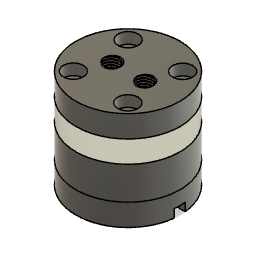
main_sensor_holder (Autodesk Fusion 360 design; units mm, degrees)
Autodesk Fusion 360 part; units mm, degrees
sketch "body_sketch" plane through (0, 0, 0) normal (0, 1, 0) x (1, 0, 0)
  circle A0 centre (0, 0) radius 19
  circle A1 centre (0, 0) radius 9.25
  circle A2 centre (0, 0) radius 14.125 construction
  circle A3 centre (9.9532, -10.0225) radius 1.65
  circle A4 centre (10.0225, 9.9532) radius 1.65
  circle A5 centre (-9.9532, 10.0225) radius 1.65
  circle A6 centre (-10.0225, -9.9532) radius 1.65
  circle A7 centre (0, 0) radius 8.25
  circle A8 centre (0, 0) radius 9.15
  circle A9 centre (9.9532, -10.0225) radius 2.1
  circle A10 centre (10.0225, 9.9532) radius 2.1
  circle A11 centre (-9.9532, 10.0225) radius 2.1
  circle A12 centre (-10.0225, -9.9532) radius 2.1
  dimension "screws_ring_dia" = 28.25
  dimension "body_dia" = 38
  dimension "sensor_cavity_dia" = 18.5
  dimension "screw_thread_hole_dia" = 3.3
  dimension "d12" = 360
  dimension "sensor_rim_min_dia" = 16.5
  dimension "sensor_holding_cylinder_clearance" = 18.3
  dimension "screw_through_hole_dia" = 4.2
  dimension "d70" = 360
  constraint coincident A0.centre A1.centre
  constraint concentric A0 A2
  constraint coincident A2 A3.centre
  constraint concentric A1 A7
  constraint concentric A1 A8
  constraint concentric A3 A9
  measures "screws_ring_dia" diameter of A2
  measures "body_dia" diameter of A0
  measures "sensor_cavity_dia" diameter of A1
  measures "screw_thread_hole_dia" diameter of A3
  measures "sensor_rim_min_dia" diameter of A7
  measures "sensor_holding_cylinder_clearance" diameter of A8
  measures "screw_through_hole_dia" diameter of A9
extrude "Extrude1" add sketch "body_sketch" along normal blind 12 contours A0 | A9 | A10 | A11 | A12 makes body 1
ref_plane "WorkPlane1" through (0, 12, 0) normal (0, 1, 0) x (1, 0, 0)
sketch " ptfe_disc_sketch_sensor_side" plane through (0, 12, 0) normal (0, 1, 0) x (1, 0, 0)
  circle A0 centre (0, 0) radius 2
  circle A1 centre (-9.9532, 10.0225) radius 2.1
  circle A2 centre (0, 0) radius 9.25
  circle A3 centre (0, 0) radius 19
  circle A4 centre (0, 0) radius 2.5 construction
  circle A5 centre (2.5, 0) radius 0.5
  circle A6 centre (-2.5, 0) radius 0.5
  line L0 (-9.9532, 10.0225) -> (10.3055, -10.3772) construction
  line L1 (0, 0) -> (-2.5, 0) construction
  circle A7 centre (0, 0) radius 14.125 construction
  circle A8 centre (-10.0225, -9.9532) radius 2.1
  circle A9 centre (9.9532, -10.0225) radius 2.1
  circle A10 centre (10.0225, 9.9532) radius 2.1
  point P0 (-9.9532, 10.0225)
  dimension "fluid_chann_intern_dist" = 5
  dimension "fluid_channel_dia" = 1
  dimension "d23" = 360
  dimension "d28" = 360
  dimension "PTFE_disc_screw_hole_dia" = 4.2
  constraint coincident A0.centre A2.centre
  constraint coincident A4 A5.centre
  constraint coincident P0 A1.centre
  constraint coincident A6.centre L1.end
  constraint concentric A0 A7
  measures "fluid_chann_intern_dist" diameter of A4
  measures "fluid_channel_dia" diameter of A5
  measures "PTFE_disc_screw_hole_dia" diameter of A1
extrude "Extrude3" add sketch " ptfe_disc_sketch_sensor_side" along normal blind 8 separate body contours A0 | A6 | A5 | A2 | A3 makes body 2
ref_plane "WorkPlane2" through (0, 20, 0) normal (0, 1, 0) x (1, 0, 0)
sketch "ptfe_disc_inlet_side" plane through (0, 20, 0) normal (0, 1, 0) x (1, 0, 0)
  circle A0 centre (0, 0) radius 6 construction
  circle A1 centre (-6, 0) radius 0.5
  circle A2 centre (6, 0) radius 0.5
  circle A3 centre (0, 0) radius 19
  circle A4 centre (-9.9532, 10.0225) radius 2.1
  circle A5 centre (-10.0225, -9.9532) radius 2.1
  circle A6 centre (9.9532, -10.0225) radius 2.1
  circle A7 centre (10.0225, 9.9532) radius 2.1
  circle A8 centre (-6, 0) radius 2
  circle A9 centre (6, 0) radius 2
  point P0 (-2.5, 0)
  point P1 (2.5, 0)
  point P2 (-9.9532, 10.0225)
  point P3 (-10.0225, -9.9532)
  point P4 (10.3055, -10.3772)
  point P5 (10.0225, 9.9532)
  dimension "fluid_channel_dia_inlet" = 1
  dimension "d35" = 360
  dimension "fluid_channel_inlet_dist" = 12
  dimension "d37" = 4.2
  dimension "d39" = 360
  dimension "fluidid_connectors_dia" = 4
  dimension "d42" = 360
  constraint coincident A0.centre A3.centre
  constraint coincident A0 A1.centre
  constraint collinear P0 A0.centre A1.centre
  constraint coincident P2 A4.centre
  constraint concentric A1 A8
  measures "fluid_channel_dia_inlet" diameter of A1
  measures "fluid_channel_inlet_dist" diameter of A0
  measures "d37" diameter of A4
  measures "fluidid_connectors_dia" diameter of A8
loft "Loft1" cut profiles " ptfe_disc_sketch_sensor_side", "ptfe_disc_inlet_side" section 1 contours A6 section 2 contours A1 bodies 2
loft "Loft2" cut profiles " ptfe_disc_sketch_sensor_side", "ptfe_disc_inlet_side" section 1 contours A5 section 2 contours A2 bodies 2
extrude "Extrude4" add sketch "ptfe_disc_inlet_side" along normal blind 8 separate body contours A3 makes body 3
copy_body "Body->Comp1" bodies 2 removing the originals makes body 4 in component "PTFE_disc"
copy_body "Body->Comp2" bodies 3 removing the originals makes body 5 in component "top_holder"
extrude "Extrude1'" add sketch "body_sketch" against normal blind 8 separate body contours A0 | A1 | A8 makes body 6 in component "bottom_sensor_holder"
extrude "Extrude3'" add sketch "body_sketch" along normal blind 4.8 contours A8 bodies 6 in component "bottom_sensor_holder"
ref_plane "WorkPlane4" through (0, 28, 0) normal (0, 1, 0) x (1, 0, 0)
sketch "top_face_sketch" plane through (0, 28, 0) normal (0, 1, 0) x (1, 0, 0)
  circle A0 centre (0, 0) radius 19
  circle A1 centre (-9.9532, 10.0225) radius 3.65
  circle A2 centre (-10.0225, -9.9532) radius 3.65
  circle A3 centre (9.9532, -10.0225) radius 3.65
  circle A4 centre (10.0225, 9.9532) radius 3.65
  point P0 (-9.9532, 10.0225)
  point P1 (10.0225, 9.9532)
  point P2 (9.9532, -10.0225)
  point P3 (-10.0225, -9.9532)
  dimension "screw_head_counter_bore" = 7.3
  dimension "d65" = 360
  constraint coincident P0 A1.centre
  measures "screw_head_counter_bore" diameter of A1
extrude "Extrude1''" cut sketch "top_face_sketch" against normal blind 4 contours A1 | A2 | A3 | A4 bodies 5 in component "top_holder"
ref_plane "WorkPlane5" through (0, -8, 0) normal (0, -1, 0) x (-1, 0, 0)
sketch "bottom_face_sketch" plane through (0, -8, 0) normal (0, -1, 0) x (1, 0, 0)
  circle A0 centre (9.9532, 10.0225) radius 2.1
  circle A1 centre (10.0225, -9.9532) radius 2.1
  circle A2 centre (-10.0225, 9.9532) radius 2.1
  circle A3 centre (-9.9532, -10.0225) radius 2.1
  circle A4 centre (0, 0) radius 8.25
  circle A5 centre (0, 0) radius 19
  circle A6 centre (-10.0225, 9.9532) radius 3.65
  circle A7 centre (-9.9532, -10.0225) radius 3.65
  circle A8 centre (10.0225, -9.9532) radius 3.65
  circle A9 centre (9.9532, 10.0225) radius 3.65
  line L0 (10.0225, -9.9532) -> (-9.9532, -10.0225) construction
  line L1 (-10.0225, 9.9532) -> (9.9532, 10.0225) construction
  circle A10 centre (-0.0473, 13.6249) radius 1.25
  line L2 (-0.0659, 18.9999) -> (-0.0286, 8.25) construction
  line L3 (-0.0473, 13.6249) -> (-10.0225, 9.9532) construction
  line L4 (-0.0473, 13.6249) -> (9.9532, 10.0225) construction
  circle A11 centre (-13.6249, -0.0473) radius 1.25
  line L5 (8.0039, -2) -> (18.8944, -2)
  line L6 (0, 0) -> (19, 0) construction
  line L7 (8.0039, 2) -> (18.8944, 2)
  circle A12 centre (0.0473, -13.6249) radius 1.25
  circle A13 centre (13.6249, 0.0473) radius 1.25
  point P0 (-10.0225, 9.9532)
  point P1 (-9.9532, -10.0225)
  point P2 (10.0225, -9.9532)
  point P3 (9.9532, 10.0225)
  dimension "screw_head_bore_bottom_dia" = 7.3
  dimension "d74" = 360
  dimension "mounting_screw_thread_hole" = 2.5
  dimension "d81" = 360
  dimension "cable_channel_width" = 2
  constraint coincident P0 A2.centre
  constraint coincident A1.centre A8.centre
  constraint coincident P1 A3.centre
  constraint coincident P3 A0.centre
  constraint coincident A10.centre L2
  constraint perpendicular L1 L2
  constraint coincident A10.centre L3.start
  constraint equal L3 L4
  constraint coincident A5 L2.start
  constraint coincident A4 L2.end
  constraint midpoint A10.centre L2
  constraint horizontal L5
  constraint coincident A4.centre A5.centre
  constraint coincident A5 L6.end
  constraint horizontal L6
  constraint symmetric L5.end L6 L7.end
  constraint symmetric L5.start L6 L7.start
  constraint coincident A4 L5.start
  constraint coincident A5 L5.end
  measures "screw_head_bore_bottom_dia" diameter of A6
  measures "mounting_screw_thread_hole" diameter of A10
  measures "cable_channel_width" distance of L5 L6
extrude "Extrude4'" cut sketch "bottom_face_sketch" against normal blind 4.6 contours A6 | A7 | A8 | A9 bodies 6 in component "bottom_sensor_holder"
extrude "Extrude5" cut sketch "bottom_face_sketch" against normal blind 3 contours A4 A5 L5 L7 | A13 picked at (13.4766, -1.7331) bodies 6 in component "bottom_sensor_holder"
extrude "Extrude6" cut sketch "bottom_face_sketch" against normal blind 8 contours A10 | A11 | A12 bodies 6 in component "bottom_sensor_holder"
thread "Thread1" "ANSI Unified Screw Threads 0.25 1/4-28 UNF 1B" major diameter 6.35 minor diameter 5.4737 pitch 0.9071 angle 60 modelled right hand crest width 0.2395 on face at (-4.0099, 22.6667, 0.1991) crest through (-3.2632, 20.2268, 0) on face at (7.9901, 22.6667, 0.1991) crest through (8.7369, 20.2268, 0) on bodies 5 in component "top_holder"
thread "Thread1'" "ISO Metric profile 4.0 M4x0.7 6H" major diameter 4.1095 minor diameter 3.332 pitch 0.7 angle 60 modelled right hand crest width 0.193 on face at (-8.3745, 8, 10.0354) crest through (-8.3565, 0.175, 9.9532) on face at (11.6011, 8, 10.1047) crest through (11.6192, 0.175, 10.0225) on face at (11.6704, 8, -9.8709) crest through (11.6885, 0.175, -9.9532) on face at (-8.3052, 8, -9.9402) crest through (-8.2872, 0.175, -10.0225) on bodies 1
thread "Thread1''" "ISO Metric profile 3.0 M3x0.5 6H" major diameter 3.086 minor diameter 2.529 pitch 0.5 angle 60 modelled right hand crest width 0.1368 on face at (1.1965, -2.6667, 13.5005) crest through (1.2172, -7.875, 13.6249) on face at (-12.3811, -2.6667, -0.1717) crest through (-13.6249, -7.875, 1.2172) on face at (1.291, -2.6667, -13.7494) crest through (1.3118, -7.875, -13.6249) on bodies 6 in component "bottom_sensor_holder"
ref_plane "WorkPlane1" through (0, 12, 0) normal (0, -1, 0) x (-1, 0, 0) in component "centering_ring"
sketch "Sketch1" plane through (0, 12, 0) normal (0, -1, 0) x (1, 0, 0) in component "centering_ring"
  circle A0 centre (0, 0) radius 9.25
  circle A1 centre (0, 0) radius 9.15
  circle A2 centre (0, 0) radius 7.25
  dimension "centering_ring_outside_dia" = 18.3
  dimension "centering_ring_inside_dia" = 14.5
  constraint concentric A0 A1
  constraint concentric A0 A2
  measures "centering_ring_outside_dia" diameter of A1
  measures "centering_ring_inside_dia" diameter of A2
extrude "Extrude1'''" add sketch "Sketch1" along normal blind 0.8 separate body contours A1 makes body 7 in component "centering_ring"
ref_plane "WorkPlane1" through (-0.0528, -8, 0) normal (0, -1, 0) x (-1, 0, 0) in component "holding_plate"
sketch "Sketch1 (2)" plane through (-0.0528, -8, 0) normal (0, -1, 0) x (1, 0, 0) in component "holding_plate"
  circle A0 centre (0.0528, 0) radius 19
  circle A1 centre (0.0528, 0) radius 8.25
  circle A2 centre (0.1, -13.6249) radius 1.25
  circle A3 centre (0.0055, 13.6249) radius 1.25
  circle A4 centre (-13.5721, -0.0473) radius 1.25
  line L0 (8.0567, -2) -> (18.9472, -2)
  line L1 (8.0567, 2) -> (18.9472, 2)
  line L2 (0, -25) -> (0.0528, 26.3634) construction
  line L3 (28, 0) -> (-44, 0) construction
  line L4 (0.0062, -18.9999) -> (-39.9938, -18.9999)
  line L5 (-39.9938, -18.9999) -> (-39.9938, 19.0001)
  line L6 (-39.9938, 19.0001) -> (0.0062, 19.0001)
  line L7 (0.0062, 19.0001) -> (0.0062, -18.9999)
  ellipse E0 centre (0.0528, 0) end of major axis (0.0062, -18.9999) minor radius 19
  line L8 (0.0994, 18.9999) -> (0.0062, -18.9999) construction
  line L9 (-18.9472, 0.0466) -> (19.0527, -0.0466) construction
  line L10 (-39.9938, 19.0001) -> (-38.3938, 19.0001)
  line L11 (-38.3938, 19.0001) -> (-38.3938, -18.9999)
  line L12 (-38.3938, -18.9999) -> (-39.9938, -18.9999)
  line L13 (-39.9938, -18.9999) -> (-39.9938, 19.0001)
  dimension "d93" = 40
  dimension "d94" = 38
  dimension "d95" = 1.6
  constraint horizontal L3
  constraint horizontal L4
  constraint vertical L5
  constraint horizontal L6
  constraint vertical L7
  constraint coincident A0 L4.start
  constraint coincident L2 L4.start
  constraint coincident E0 L8.start
  constraint coincident L4.start E0
  constraint coincident E0 L9.start
  constraint coincident E0 L9.end
  constraint concentric A0 E0
  constraint horizontal L10
  constraint vertical L11
  constraint horizontal L12
  constraint vertical L13
  constraint coincident L4 L11.end
  measures "d93" distance of L4.start L4.end
  measures "d94" distance of L4.end L5.end
  measures "d95" distance of L5.end L10.end
ref_plane "WorkPlane1" through (-40, 0, 0) normal (1, 0, 0) x (0, 1, 0) in component "holding_plate"
sketch "Sketch2" plane through (-40, 0, 0) normal (1, 0, 0) x (0, 0, -1) in component "holding_plate"
  line L0 (-19, -8) -> (19, -8)
  line L1 (19, -8) -> (19, 12)
  line L2 (14, 17) -> (-14, 17)
  line L3 (-19, 12) -> (-19, -8)
  line L4 (-14, 17) -> (-19, 12)
  line L5 (19, 12) -> (14, 17)
  line L6 (-19, -8) -> (19, -8)
  line L7 (18.9999, -8) -> (-19.0001, -8)
  line L8 (0, 19) -> (0, -14) construction
  line L9 (-22, 5) -> (23, 5) construction
  line L10 (-13, 13) -> (-5, 13)
  line L11 (-5, 13) -> (-5, 9)
  line L12 (-5, 9) -> (-13, 9)
  line L13 (-13, 9) -> (-13, 13)
  circle A0 centre (-13, 11) radius 2
  circle A1 centre (-5, 11) radius 2
  circle A2 centre (13, 11) radius 2
  circle A3 centre (5, 11) radius 2
  line L14 (13, 13) -> (5, 13)
  line L15 (5, 13) -> (5, 9)
  line L16 (13, 9) -> (13, 13)
  line L17 (5, 9) -> (13, 9)
  line L18 (5, 1) -> (13, 1)
  line L19 (-13, 1) -> (-13, -3)
  circle A4 centre (-13, -1) radius 2
  circle A5 centre (5, -1) radius 2
  line L20 (13, -3) -> (5, -3)
  circle A6 centre (13, -1) radius 2
  line L21 (13, 1) -> (13, -3)
  circle A7 centre (-5, -1) radius 2
  line L22 (-13, -3) -> (-5, -3)
  line L23 (-5, 1) -> (-13, 1)
  line L24 (5, -3) -> (5, 1)
  line L25 (-5, -3) -> (-5, 1)
  point P0 (19, 17)
  point P1 (-19, 17)
  dimension "d98" = 5
  dimension "d99" = 5
  dimension "d100" = 5
  dimension "d101" = 5
  dimension "d102" = 25
  dimension "d112" = 12
  dimension "d117" = 4
  dimension "d118" = 8
  dimension "d119" = 6
  dimension "d120" = 6
  constraint horizontal L0
  constraint vertical L1
  constraint horizontal L2
  constraint vertical L3
  constraint coincident P1 L2
  constraint coincident P1 L3
  constraint coincident P0 L1
  constraint coincident P0 L2
  constraint equal L0 L6
  constraint coincident L0.start L3.end
  constraint perpendicular L2 L8
  constraint horizontal L9
  constraint horizontal L10
  constraint vertical L11
  constraint horizontal L12
  constraint vertical L13
  constraint coincident L12.end A0
  constraint tangent L12 A0
  constraint coincident L10.start A0
  constraint coincident L11.end A1
  constraint tangent L12 A1
  constraint coincident L10.end A1
  constraint symmetric L8 L10.start L14.start
  constraint symmetric L8 L10.end L14.end
  constraint symmetric L8 L11.end L15.end
  constraint symmetric L8 L12.end L16.start
  constraint symmetric L8 A0 A2
  constraint symmetric L8 A1 A3
  constraint symmetric L9 L10.start L19.end
  constraint symmetric L9 L10.end L22.end
  constraint symmetric L9 L11.end L23.start
  constraint symmetric L9 L12.end L19.start
  constraint symmetric L9 A0 A4
  constraint symmetric L9 A1 A7
  constraint symmetric L9 A2 A6
  constraint symmetric L9 A3 A5
  constraint symmetric L9 L14.start L20.start
  constraint symmetric L9 L14.end L20.end
  constraint symmetric L9 L15.end L18.start
  constraint symmetric L9 L16.start L18.end
  measures "d98" distance of P1 L2.end
  measures "d99" distance of P1 L3.start
  measures "d100" distance of P0 L1.end
  measures "d101" distance of P0 L2.start
  measures "d102" distance of L2 L6
  measures "d112" distance of L2 L9
  measures "d117" distance of L10 L12
  measures "d118" distance of L11 L13
  measures "d119" distance of L2 A0.centre
  measures "d120" distance of L3 A0.centre
extrude "Extrude1''''" add sketch "Sketch1 (2)" along normal blind 1.6 separate body contours A0 A1 L0 L1 E0 | A0 A1 A3 L1 L7 E0 | A0 A1 A2 L0 L7 E0 | A0 A1 A2 A3 L7 E0 | A0 L4 L6 E0 L11 | A1 L7 | L4 L5 L6 L10 L11 L12 L13 | A1 L7 makes body 8 in component "holding_plate"
extrude "Extrude2" add sketch "Sketch2" along normal blind 1.6 bodies 8 in component "holding_plate"
component "bottom_sensor_holder" placed x (1, 0, 0) y (0, 1, 0) z (0, 0, 1) at (0, 0, 0)
component "PTFE_disc" placed x (1, 0, 0) y (0, 1, 0) z (0, 0, 1) at (0, 0, 0)
component "top_holder" placed x (1, 0, 0) y (0, 1, 0) z (0, 0, 1) at (0, 0, 0)
component "centering_ring" placed x (1, 0, 0) y (0, 1, 0) z (0, 0, 1) at (0, 0, 0)
component "holding_plate" placed x (1, 0, 0) y (0, 1, 0) z (0, 0, 1) at (0, 0, 0)
equation "screws_ring_dia = 1 / 2 * ( body_dia + sensor_cavity_dia )"
equation "Body_height = 12.00 mm"
equation "ptfe_bottom_plane_dist = 0.00 mm"
equation "PTFE_disc_screw_hole_dia = screw_through_hole_dia"
equation "ptfe_thickness = 8.00 mm"
equation "ptfe_top_plane_dist = ptfe_bottom_plane_dist"
equation "fluid_channel_dia_inlet = fluid_channel_dia"
equation "fluid_channel_inlet_dist = fluid_chann_intern_dist + 7 mm"
equation "d37 = PTFE_disc_screw_hole_dia"
equation "top_holder_thickness = 8.00 mm"
equation "bottom_holder_thickness = -8.00 mm"
equation "MPS_holding_cylinder = Body_height - MPS_thickness - 1 / 2 * o_ring_thickness"
equation "MPS_thickness = 6.7 mm"
equation "o_ring_thickness = 1 mm"
equation "sensor_holding_cylinder_clearance = sensor_cavity_dia - 0.2 mm"
equation "screw_head_hole_depth = -4.00 mm"
equation "screw_head_bore_bottom_dia = screw_head_counter_bore"
equation "screw_head_bottom_hole_depth = -4.60 mm"
equation "cable_channel_depth = -3 mm"
equation "mounting_screw_threaded_hole_depth = bottom_holder_thickness"
equation "centering_ring_outside_dia = sensor_cavity_dia - 0.2 mm"
equation "centering_ring_height = 0.80 mm"
equation "d94 = body_dia"
equation "d99 = d98"
equation "d101 = d100"
named bodies: "holder_body", "PTFE_disc", "top_holder", "bottom_sensor_holder"
